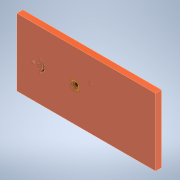
# Autodesk Inventor part: Cover
Saved by Autodesk Inventor 2022.2 (Build 262287010, 287A)
## iProperties
Created: 2022-03-17
Part Number: Cover
Material: Genérico
Document SubType Name: Modeling
Designer: mabel
Density: 1 g/cm^3
Appearance: Suave - Naranja claro
Author: mabel
Autodesk Inventor part; units mm, degrees
ref_plane "YZ Plane" through (0, 0, 0) normal (1, 0, 0) x (0, 1, 0)
ref_plane "XZ Plane" through (0, 0, 0) normal (0, 1, 0) x (-1, 0, 0)
sketch "Boceto2" plane through (0, 0, 0) normal (0, 0, 1) x (1, 0, 0)
  line L0 (130, -85) -> (-130, -85)
  line L1 (-130, -85) -> (-130, 85)
  line L2 (-130, 85) -> (130, 85)
  line L3 (130, 85) -> (130, -85)
  line L4 (130, -85) -> (-130, 85) construction
  line L5 (-130, -85) -> (130, 85) construction
  point P0 (0, 0)
  dimension "d0" = 260
  dimension "d1" = 170
  constraints: 12 end point, 2 midpoint, 2 parallel, 1 horizontal, 1 perpendicular
  measures "d0" distance of L1.end L2.end
  measures "d1" distance of L0.end L1.end
extrude "Extrusión1" add sketch "Boceto2" along normal blind 15
sketch "Boceto3" plane through (0, 0, 15) normal (0, 0, 1) x (1, 0, 0)
  line L0 (-95, 0) -> (-4.19, 0) construction
  circle A0 centre (-95, 0) radius 2.625
  circle A1 centre (-4.19, 0) radius 9.875
  line L1 (-130, 85) -> (-130, -85) projected
  line L2 (130, -85) -> (130, 85) projected
  line L3 (-130, -85) -> (130, -85) projected
  line L4 (130, 0) -> (80, 0) construction
  line L5 (80, 0) -> (80, -23.2237) construction
  arc A2 (-102.5, -15.9496) -> (-102.5, 15.9496) centre (-109.9995, 0) ccw
  arc A3 (-102.5, -9.8973) -> (-102.5, 9.8973) centre (-109.9995, 0) ccw
  line L6 (-95, 0) -> (-102.5, 0)
  line L7 (-102.5, 15.9496) -> (-102.5, 12.8966)
  line L8 (-102.5, 15.9496) -> (-102.5, 9.8973)
  line L9 (-102.5, -9.8973) -> (-102.5, -15.9496)
  point P0 (0, 0)
  point P1 (-130, 0)
  point P2 (-92.375, 0)
  point P3 (-97.5893, -0.4312)
  point P4 (-97.5893, 0.4312)
  dimension "d7" = 5.25
  dimension "d8" = 19.75
  dimension "d14" = 85
  dimension "d29" = 50
  dimension "d31" = 35
  dimension "d32" = 134.19
  dimension "d139" = 125.81
  dimension "d141" = 7.5
  constraints: 14 end point, 4 centre point, 4 point on circle, 3 coincident, 3 horizontal, 2 midpoint, 2 vertical, 1 perpendicular
  measures "d7" diameter of A0
  measures "d8" diameter of A1
  measures "d14" distance from line of L3 L0.end
  measures "d29" distance of L4.start L4.end
  measures "d31" distance from line of L6.start L1
  measures "d32" distance from line of L2 A1.centre
  measures "d139" distance from line of L0.end L1
  measures "d141" distance of L6.start L6.end
sketch "Boceto5" plane through (0, 0, 0) normal (0, 0, -1) x (-1, 0, 0)
  line L0 (-130, -85) -> (-130, 85) projected
  line L1 (130, -85) -> (-130, -85)
  line L2 (-130, -85) -> (-130, 85)
  line L3 (-130, 85) -> (130, 85)
  line L4 (130, 85) -> (130, -85)
  line L5 (130, -85) -> (-130, 85) construction
  line L6 (-130, -85) -> (130, 85) construction
  line L7 (119.5, 74.5) -> (-119.5, 74.5)
  line L8 (-119.5, 74.5) -> (-119.5, -74.5)
  line L9 (-119.5, -74.5) -> (119.5, -74.5)
  line L10 (119.5, -74.5) -> (119.5, 74.5)
  circle A0 centre (95, 0) radius 2.625 projected
  circle A1 centre (95, 0) radius 2.625
  point P0 (0, 0)
  dimension "d23" = 10.5
  dimension "d25" = 5.25
  constraints: 20 end point, 4 parallel, 2 midpoint, 2 perpendicular, 1 centre point, 1 coincident, 1 horizontal, 3 other
  measures "d23" distance between parallel lines of L3 L7
  measures "d25" diameter of A1
sketch "Boceto6" plane through (0, 0, 15) normal (0, 0, 1) x (1, 0, 0)
  circle A0 centre (-4.19, 0) radius 10.125 projected
  line L0 (-4.19, 0) -> (35.81, 0)
  line L1 (35.81, 0) -> (35.81, 25)
  circle A1 centre (35.81, 25) radius 2.5
  point P0 (0, 0)
  dimension "d35" = 40
  dimension "d36" = 25
  dimension "d152" = 5
  constraints: 4 end point, 1 centre point, 1 coincident, 1 horizontal, 1 perpendicular
  measures "d35" distance of L0.start L0.end
  measures "d36" distance of L0.end L1.end
  measures "d152" diameter of A1
ref_plane "Plano de trabajo4" through (0, 0, -4) normal (0, 0, -1) x (-1, 0, 0)
sketch "Boceto10" plane through (0, 0, -4) normal (0, 0, -1) x (-1, 0, 0)
  circle A0 centre (95, 0) radius 2.625 projected
  circle A1 centre (95, 0) radius 7.5
  point P0 (0, 0)
  dimension "d51" = 15
  constraints: 1 centre point, 1 coincident
  measures "d51" diameter of A1
ref_plane "Plano de trabajo1" through (-95, 0, 0) normal (0, 0, -1) x (-1, 0, 0)
sketch "Boceto12" plane through (0, 0, 15) normal (0, 0, 1) x (1, 0, 0)
  circle A0 centre (-95, 0) radius 2.625 construction
  circle A1 centre (-95, 0) radius 7.5 construction
  line L0 (-95, 0) -> (-82.5, 0) construction
  circle A2 centre (-82.5, 0) radius 3
  line L1 (-95, 0) -> (-107.5, 0) construction
  circle A3 centre (-107.5, 0) radius 3
  circle A4 centre (-107.5, 0) radius 1.5 construction
  circle A5 centre (-82.5, 0) radius 1.5 construction
  line L2 (-82.5, 0) -> (-97.5, 0) construction
  line L3 (-97.5, 0) -> (-97.5, 18.5) construction
  arc A6 (-89.1168, -15.9286) -> (-89.9998, 16.363) centre (-97.5, 0) ccw
  arc A7 (-89.9998, -16.2295) -> (-89.1168, -15.9286) centre (-90.514, -13.2739) ccw
  arc A8 (-89.9998, -16.2295) -> (-89.1168, -15.9286) centre (-90.514, -13.2739) ccw
  arc A9 (-92.595, 10.9517) -> (-92.4052, 10.8647) centre (-91.2508, 13.6338) ccw
  arc A10 (-89.9998, -16.2295) -> (-89.1168, -15.9286) centre (-90.514, -13.2739) ccw
  arc A11 (-89.8154, -14.6013) -> (-90, 14.6969) centre (-97.5, 0) ccw
  arc A12 (-89.9998, -11.2249) -> (-90, 11.225) centre (-97.5, 0) ccw
  arc A13 (-89.9998, -14.683) -> (-89.8154, -14.6013) centre (-90.514, -13.2739) ccw
  circle A14 centre (-82.5, 0) radius 1.5
  line L4 (-130, 85) -> (-130, -85) projected
  line L5 (-130, -85) -> (130, -85) projected
  line L6 (-82.5, 0) -> (-90, 0) construction
  line L7 (-90, 0) -> (-90, 18.2385) construction
  line L8 (-89.9998, 16.363) -> (-89.9998, -17.0131)
  arc A15 (-89.9998, -9.3674) -> (-90, 9.3675) centre (-97.5, 0) ccw
  arc A16 (-92.4052, 10.8647) -> (-92.6345, 10.9694) centre (-97.5, 0) ccw
  point P0 (0, 0)
  point P1 (-89.8154, -14.6013)
  point P2 (-91.2126, -11.9465)
  point P3 (-84.225, -2.4545)
  point P4 (-79.5, 0)
  point P5 (-81.225, -2.7156)
  point P6 (-84.225, 2.4545)
  point P7 (-81.225, 2.7156)
  point P8 (-84, 0)
  point P9 (-81, 0)
  point P10 (-89.9998, 11.2249)
  point P11 (-89.9998, 9.3674)
  point P12 (-85.5, 0)
  point P13 (-89.9998, 14.6969)
  dimension "d59" = 15
  dimension "d60" = 12.5
  dimension "d61" = 6
  dimension "d62" = 12.5
  dimension "d63" = 6
  dimension "d64" = 3
  dimension "d65" = 3
  dimension "d126" = 15
  dimension "d127" = 6
  dimension "d128" = 6
  dimension "d129" = 1.5
  dimension "d130" = 1.5
  dimension "d135" = 3
  constraints: 21 point on circle, 16 centre point, 14 end point, 8 coincident, 8 point on line, 3 vertical, 2 horizontal, 1 midpoint, 1 tangent
  measures "d59" diameter of A1
  measures "d60" distance of L0.start L0.end
  measures "d61" diameter of A2
  measures "d62" distance of L0.start L1.end
  measures "d63" diameter of A3
  measures "d64" diameter of A4
  measures "d65" diameter of A5
  measures "d126" distance of L2.start L2.end
  measures "d127" diameter of A9
  measures "d128" diameter of A10
  measures "d129" radial gap between concentric circles of A6 A11
  measures "d130" radial gap between concentric circles of A10 A13
  measures "d135" diameter of A14
extrude "Extrusión10" cut sketch "Boceto12" against normal blind 1.5 contours A2 A11 | A11 A14 A12 A2 | A2 A12 A14 A11 | A12 A2 | A14 | A3
sketch "Boceto13" plane through (-82.5, 0, 13.5) normal (0, 0, 1) x (1, 0, 0)
  circle A0 centre (0, 0) radius 1.5
  circle A1 centre (-25, 0) radius 3 projected
  circle A2 centre (-25, 0) radius 1.5
  point P0 (82.5, 0)
  dimension "d68" = 3
  dimension "d69" = 3
  constraints: 2 centre point, 1 coincident
  measures "d68" diameter of A0
  measures "d69" diameter of A2
extrude "Extrusión11" cut sketch "Boceto13" against normal through all contours A0 | A2
extrude "Extrusión12" cut sketch "Boceto10" against normal blind 5
ref_plane "Plano de trabajo2" through (-4.19, 0, 15) normal (0, 0, 1) x (1, 0, 0)
sketch "Boceto15" plane through (-4.19, 0, 15) normal (0, 0, 1) x (1, 0, 0)
  circle A0 centre (0, 0) radius 5
  circle A1 centre (0, 0) radius 74 construction
  circle A2 centre (-90.81, 0) radius 2.625 construction
  circle A3 centre (-90.81, 0) radius 20 construction
  point P0 (4.19, 0)
  dimension "d77" = 10
  dimension "d80" = 148
  dimension "d82" = 40
  constraints: 3 centre point, 2 coincident
  measures "d77" diameter of A0
  measures "d80" diameter of A1
  measures "d82" diameter of A3
extrude "Extrusión14" cut sketch "Boceto15" against normal through all
ref_plane "Plano de trabajo3" through (0, 0, -4) normal (0, 0, -1) x (-1, 0, 0)
sketch "Boceto17" plane through (0, 0, 15) normal (0, 0, 1) x (1, 0, 0)
  circle A0 centre (-95, 0) radius 2.625 construction
  circle A1 centre (-4.19, 0) radius 5 construction
  circle A2 centre (-4.19, 0) radius 40
  circle A3 centre (-4.19, 0) radius 15
  point P0 (0, 0)
  dimension "d87" = 80
  dimension "d88" = 30
  constraints: 2 centre point, 2 coincident
  measures "d87" diameter of A2
  measures "d88" diameter of A3
sketch "Boceto20" plane through (0, 0, 15) normal (0, 0, 1) x (1, 0, 0)
  line L0 (130, 85) -> (-130, 85) projected
  line L1 (130, -85) -> (130, 85)
  line L2 (130, 85) -> (220, 85)
  line L3 (220, 85) -> (220, -85)
  line L4 (220, -85) -> (130, -85)
  line L5 (130, -85) -> (130, 85)
  point P0 (0, 0)
  dimension "d115" = 90
  constraints: 10 end point, 2 parallel, 1 horizontal, 1 perpendicular
  measures "d115" distance of L3.end L4.end
extrude "Extrusión22" add sketch "Boceto20" against normal blind 15
extrude "Extrusión23" cut sketch "Boceto3" against normal through all contours A0 A3 | A3 L6 A0 | A0 L6 A3
extrude "Extrusión24" [suppressed]
extrude "Extrusión25" cut sketch "Boceto12" against normal blind 1.5 contours A2 A11 | A6 A7 L8 A13 A11 A2 | A2 A11 L8 A6 | A12 A2 | A2 A15 L8 A12 | A12 L8 A15 A2
extrude "Extrusión26" cut sketch "Boceto12" against normal through all contours A11 A14 A12 A2 | A2 A12 L8 A11 | A11 A13 L8 A12 A2 | A2 A12 A14 A11
sketch "Boceto21" plane through (0, 0, 15) normal (0, 0, 1) x (1, 0, 0)
  line L0 (-130, 85) -> (-150, 85)
  line L1 (-150, 85) -> (-150, -85)
  line L2 (-150, -85) -> (-130, -85)
  line L3 (-130, -85) -> (-130, 85)
  line L4 (220, 85) -> (-130, 85) projected
  line L5 (-130, -85) -> (220, -85) projected
  line L6 (220, 85) -> (200, 85)
  line L7 (200, 85) -> (200, -85)
  line L8 (200, -85) -> (220, -85)
  line L9 (220, -85) -> (220, 85)
  point P0 (0, 0)
  dimension "d146" = 20
  dimension "d147" = 20
  constraints: 16 end point, 4 parallel, 2 horizontal, 2 perpendicular, 1 point on line
  measures "d146" distance of L2.end L1.end
  measures "d147" distance of L8.end L7.end
extrude "Extrusión28" add sketch "Boceto21" against normal blind 15 contours L3 L2 L1 L0
extrude "Extrusión29" cut sketch "Boceto21" against normal through all contours L4 L9 L5 L7
extrude "Extrusión30" cut sketch "Boceto6" against normal through all contours A1
extrude "Extrusión31" cut sketch "Boceto3" against normal blind 3.5 contours A1
